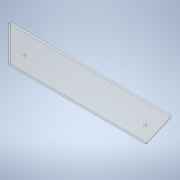
# Autodesk Inventor part: UpperAcrylicSheetSide
Saved by Autodesk Inventor 2021 (Build 250183000, 183)
## iProperties
Created: 2020-07-17
Part Number: UpperAcrylicSheetSide
Material: Generic
Document SubType Name: Modeling
Designer: CASE-SMALL2
Density: 1 g/cm^3
Appearance: Default
Author: CASE-SMALL2
Autodesk Inventor part; units mm, degrees
ref_plane "YZ Plane" through (0, 0, 0) normal (1, 0, 0) x (0, 1, 0)
ref_plane "XZ Plane" through (0, 0, 0) normal (0, 1, 0) x (-1, 0, 0)
ref_plane "XY Plane" through (0, 0, 0) normal (0, 0, 1) x (1, 0, 0)
sketch "Sketch1" plane through (0, 0, 0) normal (0, 0, 1) x (1, 0, 0)
  line L0 (-134.5, -30) -> (134.5, -30)
  line L1 (134.5, -30) -> (134.5, 30)
  line L2 (134.5, 30) -> (-134.5, 30)
  line L3 (-134.5, 30) -> (-134.5, -30)
  line L4 (-134.5, -30) -> (134.5, 30) construction
  line L5 (134.5, -30) -> (-134.5, 30) construction
  line L6 (134.5, 30) -> (92.4875, -30)
  point P0 (0, 0)
  dimension "d0" = 269
  dimension "d1" = 60
  dimension "d2" = 55
  constraints: 14 end point, 2 midpoint, 2 parallel, 1 horizontal, 1 perpendicular, 1 point on line
  measures "d0" distance of L1.end L2.end
  measures "d1" distance of L0.end L1.end
  measures "d2" angle of L0 L6
extrude "Extrusion1" add sketch "Sketch1" along normal blind 3 contours L3 L2 L6 L0
sketch "Sketch2" plane through (0, 0, 3) normal (0, 0, 1) x (1, 0, 0)
  circle A0 centre (-109.5, -5) radius 1.65
  line L0 (-134.5, -30) -> (92.4875, -30) projected
  line L1 (-134.5, 30) -> (-134.5, -30) projected
  line L2 (-109.5, -5) -> (151.1099, -5) construction
  circle A1 centre (90.5, -5) radius 1.65
  point P0 (0, 0)
  dimension "d5" = 25
  dimension "d6" = 3.3
  dimension "d7" = 25
  dimension "d8" = 225
  dimension "d9" = 3.3
  constraints: 2 centre point, 2 end point, 1 horizontal, 1 point on line
  measures "d5" distance from line of L0 L2.start
  measures "d6" diameter of A0
  measures "d7" distance from line of L1 L2.start
  measures "d8" distance from line of A1.centre L1
  measures "d9" diameter of A1
extrude "Extrusion2" cut sketch "Sketch2" against normal through all
fillet "Fillet1" radius 2 4 edges at (-134.5, 30, 1.5) (-134.5, -30, 1.5) (92.4875, -30, 1.5) (134.5, 30, 1.5)
sketch "Sketch3" plane through (0, 0, 3) normal (0, 0, 1) x (1, 0, 0)
  arc A0 (132.2963, 26.8528) -> (130.658, 30) centre (130.658, 28) ccw projected
  line L0 (130.658, 30) -> (-132.5, 30) projected
  arc A1 (-132.5, 30) -> (-134.5, 28) centre (-132.5, 28) ccw projected
  line L1 (-134.5, 28) -> (-134.5, -28) projected
  arc A2 (-134.5, -28) -> (-132.5, -30) centre (-132.5, -28) ccw projected
  line L2 (-132.5, -30) -> (91.4464, -30) projected
  arc A3 (91.4464, -30) -> (93.0847, -29.1472) centre (91.4464, -28) ccw projected
  line L3 (93.0847, -29.1472) -> (132.2963, 26.8528) projected
  circle A4 centre (90.5, -5) radius 1.65 projected
  circle A5 centre (-109.5, -5) radius 1.65 projected
  point P0 (0, 0)
equation "\"d9\" = d6"
body "Solid1"
